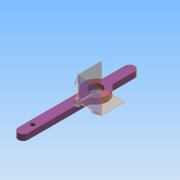
# Autodesk Inventor part: Selection_Lever 3
Saved by Autodesk Inventor 2018.1 (Build 221171000, 171)
## iProperties
Created: 2019-02-16
Part Number: Selection_Lever 3
Material: Nylon 6/6
Document SubType Name: Modeling
Designer: James
Density: 1.13 g/cm^3
Appearance: Nylon 6
Mass: 1.07509 g
Surface Area: 10.8673 cm^2
Volume: 0.951403 cm^3
Author: James
Autodesk Inventor part; units mm, degrees
ref_plane "YZ Plane" through (0, 0, 0) normal (1, 0, 0) x (0, 1, 0)
ref_plane "XZ Plane" through (0, 0, 0) normal (0, 1, 0) x (-1, 0, 0)
ref_plane "XY Plane" through (0, 0, 0) normal (0, 0, 1) x (1, 0, 0)
sketch "Sketch1" plane through (0, 0, 0) normal (0, 0, 1) x (1, 0, 0)
  line L0 (0, 0) -> (5, 0)
  line L1 (5, 0) -> (5, 60)
  line L2 (5, 60) -> (0, 60)
  line L3 (0, 60) -> (0, 0)
  circle A0 centre (2.5, 40) radius 6
  point P0 (2.5, 60)
  dimension "d0" = 5
  dimension "d1" = 60
  dimension "d14" = 12
  dimension "d15" = 20
  constraints: 8 end point, 2 parallel, 1 centre point, 1 horizontal, 1 midpoint, 1 perpendicular, 1 vertical alignment
  measures "d0" distance of L1.end L2.end
  measures "d1" distance of L0.end L1.end
  measures "d14" diameter of A0
  measures "d15" distance of point (2.5, 60) A0.centre
extrude "Extrusion1" add sketch "Sketch1" along normal blind 3
full round fillet "Fillet2" first side at (0, 23.0304, 2) centre faces at (1.6667, 0, 1) second side at (5, 11.5152, 1)
full round fillet "Fillet3" first side at (0, 55.1515, 1) centre faces at (3.3333, 60, 1) second side at (5, 50.3029, 1)
sketch "Sketch3" plane through (0, 0, 3) normal (0, 0, 1) x (1, 0, 0)
  arc A0 (5, 34.5456) -> (5, 45.4544) centre (2.5, 40) ccw projected
  point P0 (0, 0)
  constraints: 1 coincident
hole "Hole2" at (2.5, 40, 3) direction (0, 0, -1) diameter 6.5 end through all
fillet "Fillet4" radius 2 4 edges at (5, 45.4544, 1.5) (0, 45.4544, 1.5) (5, 34.5456, 1.5) (0, 34.5456, 1.5)
sketch "Sketch4" plane through (0, 0, 0) normal (0, 0, -1) x (-1, 0, 0)
  line L0 (-5, 2.5) -> (-5, 33.3856) projected
  line L1 (0, 33.3856) -> (0, 2.5) projected
  point P0 (0, 0)
  point P1 (-2.5, 7.5)
  dimension "d24" = 2.5
  dimension "d25" = 2.5
  dimension "d26" = 5
  measures "d24" distance from line of L0 point (-2.5, 7.5)
  measures "d25" distance from line of L1 point (-2.5, 7.5)
  measures "d26" vertical distance of L0.start point (-2.5, 7.5)
hole "Hole3" at (2.5, 7.5, 0) direction (0, 0, 1) diameter 2 end through all
equation "\"d24\" = d25"
body "Solid1"
